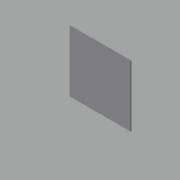
# Autodesk Inventor part: HEATBED MK3
Saved by Autodesk Inventor 2013 (Build 170138000, 138)
## iProperties
Created: 2015-04-03
Part Number: HEATBED MK3
Material: Aluminum
Document SubType Name: Modeling
Designer: Ultimate
Density: 1 g/cm^3
Author: Ultimate
Autodesk Inventor part; units mm, degrees
ref_plane "YZ Plane" through (0, 0, 0) normal (1, 0, 0) x (0, 1, 0)
ref_plane "XZ Plane" through (0, 0, 0) normal (0, 1, 0) x (-1, 0, 0)
ref_plane "XY Plane" through (0, 0, 0) normal (0, 0, 1) x (1, 0, 0)
sketch "Sketch1" plane through (0, 0, 0) normal (0, 1, 0) x (-1, 0, 0)
  line L0 (-107, 107) -> (107, 107)
  line L1 (107, 107) -> (107, -107)
  line L2 (107, -107) -> (-107, -107)
  line L3 (-107, -107) -> (-107, 107)
  line L4 (104.5, 104.5) -> (-104.5, 104.5)
  line L5 (-104.5, 104.5) -> (-104.5, -104.5)
  line L6 (-104.5, -104.5) -> (104.5, -104.5)
  line L7 (104.5, -104.5) -> (104.5, 104.5)
  line L8 (-107, 107) -> (107, 107) construction
  line L9 (107, 107) -> (107, -107) construction
  line L10 (107, -107) -> (-107, -107) construction
  line L11 (-107, -107) -> (-107, 107) construction
  point P0 (0, 0)
  dimension "d0" = 214
  dimension "d1" = 214
  dimension "d2" = 107
  dimension "d3" = 107
  dimension "d4" = 209
  dimension "d5" = 209
  dimension "d6" = 104.5
  dimension "d7" = 104.5
  constraints: 16 end point, 5 coincident, 4 parallel, 2 horizontal, 2 perpendicular, 2 other
  measures "d0" distance of L1.end L2.end
  measures "d1" distance of L0.end L1.end
  measures "d2" distance from line of L3 point (0, 0)
  measures "d3" distance from line of L0 point (0, 0)
  measures "d4" distance of L6.end L5.end
  measures "d5" distance of L5.end L4.end
  measures "d6" distance from line of point (0, 0) L5
  measures "d7" distance from line of L6 point (0, 0)
extrude "Extrusion1" add sketch "Sketch1" against normal blind 3 contours L0 L1 L2 L3 | L7 L6 L5 L4
hole "Hole1" at (104.5, 0, 104.5) at (-104.5, 0, 104.5) at (-104.5, 0, -104.5) at (104.5, 0, -104.5) direction (0, -1, 0) diameter 3 depth 8 tip angle 118
decal "Decal1"
body "Solid1"
